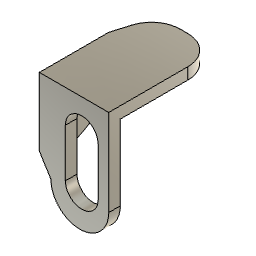
Corner safeguard (Autodesk Fusion 360 design; units mm, degrees)
Autodesk Fusion 360 part; units mm, degrees
sketch "Sketch1" plane through (0, 0, 0) normal (0, 0, 1) x (1, 0, 0)
  line L0 (0, 0) -> (15, 0)
  line L1 (15, 0) -> (15, 25)
  line L2 (15, 25) -> (0, 25)
  line L3 (0, 25) -> (0, 0)
  line L4 (0, 0) -> (15, 0)
  line L5 (15, 0) -> (15, -3)
  line L6 (15, -3) -> (0, -3)
  line L7 (0, -3) -> (0, 0)
  dimension "d1" = 15
  dimension "d2" = 25
  dimension "d3" = 3
  constraint horizontal L0
  constraint vertical L1
  constraint horizontal L2
  constraint vertical L3
  constraint coincident L0.start L3.end
  constraint horizontal L4
  constraint vertical L5
  constraint horizontal L6
  constraint vertical L7
  measures "d1" distance of L0.start L0.end
  measures "d2" distance of L0.end L1.end
  measures "d3" distance of L0.start L6.end
extrude "Extrude1" add sketch "Sketch1" along normal blind 3 contours L0 L1 L2 L3 L4
extrude "Extrude2" add sketch "Sketch1" along normal blind 30 contours L0 L4 L5 L6 L7
sketch "Sketch2" plane through (0, -3, 0) normal (0, -1, 0) x (1, 0, 0)
  line L0 (0, 0) -> (15, 0)
  line L1 (15, 0) -> (15, 30)
  line L2 (15, 30) -> (0, 30)
  line L3 (0, 30) -> (0, 0)
  circle A0 centre (7, 21) radius 4.25
  circle A1 centre (7, 8.5) radius 4.25
  line L4 (11.25, 21) -> (11.25, 8.5)
  line L5 (2.75, 21) -> (2.75, 8.5)
  dimension "d8" = 8.5
  dimension "d9" = 8.5
  dimension "d12" = 8.5
  dimension "d13" = 9
  dimension "d18" = 8
  constraint coincident A0 L4.start
  constraint coincident A1 L4.end
  constraint tangent A1 L4
  constraint coincident A0 L5.start
  constraint coincident A1 L5.end
  constraint tangent A1 L5
  constraint parallel L3 L5
  measures "d8" diameter of A0
  measures "d9" diameter of A1
  measures "d12" distance of L0 A1.centre
  measures "d13" distance of L2 A0.centre
  measures "d18" distance of L1 A1.centre
extrude "Extrude3" cut sketch "Sketch2" against normal blind 3 contours A0 | A0 A1 L4 L5 | A1
fillet "Fillet1" radius 7.5 2 edges at (15, -1.5, 30) (0, -1.5, 30)
move_body "Move1" bodies 1 to x (-1, 0, 0) y (0, 1, 0) z (0, 0, -1) at (15, 0, 31)
sketch "Sketch3" plane through (0, 0, 0) normal (-1, 0, 0) x (0, -1, 0)
  line L0 (0, 8.5) -> (3, 8.5)
  line L1 (3, 8.5) -> (3, 31)
  line L2 (3, 31) -> (-25, 31)
  line L3 (-25, 31) -> (-25, 28)
  line L4 (-25, 28) -> (0, 28)
  line L5 (0, 28) -> (0, 8.5)
  line L6 (3, 31) -> (-15, 31)
  line L7 (3, 13) -> (3, 31)
  arc A0 (-15, 31) -> (3, 13) centre (3, 31) ccw
  dimension "d21" = 18
  constraint horizontal L6
  constraint vertical L7
  constraint coincident L1.end L2.start
  constraint coincident L6.end A0.start
  constraint coincident L7.start A0.end
  measures "d21" radius of A0
extrude "Extrude4" add sketch "Sketch3" along normal blind 3 contours L4 L5 A0 | L1 L2 L4 L5 L6 L7 A0
extrude "Extrude5" add 1 faces at (0, -1.6653, 10.0083) along direction (-1, 0, 0) blind 3
chamfer "Chamfer1" distance 4.8 distance2 3 1 edges at (-3, -1.5, 8.5) measured on face at (-3, -2, 17.5834)
extrude "Extrude6" add 1 faces at (0, 21.6573, 29.6653) along direction (-1, 0, 0) blind 3
chamfer "Chamfer2" distance 10 distance2 3 1 edges at (-3, 25, 29.5) measured on face at (-3, 12.2494, 30)
fillet "Fillet2" radius 7.5 2 edges at (15, 25, 29.5) (0, 25, 29.5)
equation "d6 = 3 mm + 27 mm"
equation "d12 = 3 mm + ( 9 / 2 ) * 1 mm + 1 mm"
equation "d17 = ( 15 / 2 ) * 1 mm"
equation "d31 = ( 15 / 2 ) * 1 mm"
